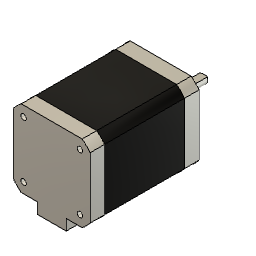
Planetary Gear Module v11 (Autodesk Fusion 360 archive; units mm, degrees)
design "Nema 17 Stepper Motor 60mm"
Autodesk Fusion 360 part; units mm, degrees
sketch "Sketch1" plane through (0, 0, 0) normal (0, 0, 1) x (1, 0, 0)
  line L0 (-15.5, 15.5) -> (15.5, 15.5) construction
  line L1 (15.5, 15.5) -> (15.5, -15.5) construction
  line L2 (15.5, -15.5) -> (-15.5, -15.5) construction
  line L3 (-15.5, -15.5) -> (-15.5, 15.5) construction
  line L4 (15.5, 15.5) -> (-15.5, -15.5) construction
  line L5 (-21.15, 21.15) -> (21.15, 21.15)
  line L6 (21.15, 21.15) -> (21.15, -21.15)
  line L7 (21.15, -21.15) -> (-21.15, -21.15)
  line L8 (-21.15, -21.15) -> (-21.15, 21.15)
  line L9 (-21.15, 21.15) -> (21.15, -21.15) construction
  arc A0 (-21.15, -16.7833) -> (-16.7833, -21.15) centre (0, 0) ccw
  arc A1 (16.7833, -21.15) -> (21.15, -16.7833) centre (0, 0) ccw
  arc A2 (21.15, 16.7833) -> (16.7833, 21.15) centre (0, 0) ccw
  arc A3 (-16.7833, 21.15) -> (-21.15, 16.7833) centre (0, 0) ccw
  circle A4 centre (0, 0) radius 11
  circle A5 centre (0, 0) radius 2.5
  line L10 (-2, 1.5) -> (2, 1.5)
  circle A6 centre (-15.5, 15.5) radius 1.5
  circle A7 centre (-15.5, -15.5) radius 1.5
  circle A8 centre (15.5, -15.5) radius 1.5
  circle A9 centre (15.5, 15.5) radius 1.5
  circle A10 centre (0, 0) radius 5
  line L11 (0, -2.5) -> (0, 1.5) construction
  line L12 (8, -21.15) -> (8, -27.15)
  line L13 (8, -27.15) -> (-8, -27.15)
  line L14 (-8, -27.15) -> (-8, -21.15)
  line L15 (0, 0) -> (0, -21.15) construction
  point P0 (0, -2.5)
  dimension "d37" = 60
  dimension "d39" = -52
  dimension "d40" = 0
  constraint horizontal L0
  constraint vertical L1
  constraint horizontal L2
  constraint vertical L3
  constraint equal L0 L3
  constraint midpoint A0.centre L4
  constraint coincident A0.centre A1.centre
  constraint horizontal L5
  constraint vertical L6
  constraint horizontal L7
  constraint vertical L8
  constraint coincident L4 L7.end
  constraint coincident L4 L5.end
  constraint coincident L8 A3.end
  constraint coincident L8 A0.start
  constraint coincident L7 A0.end
  constraint concentric A0 A1
  constraint coincident L7 A1.start
  constraint coincident L6 A1.end
  constraint coincident L6 A2.start
  constraint coincident L5 A3.start
  constraint concentric A2 A3
  constraint coincident L5 A2.end
  constraint equal A2 A3
  constraint equal A1 A3
  constraint equal A0 A3
  constraint concentric A2 A4
  constraint coincident A5 L10.start
  constraint coincident A5 L10.end
  constraint horizontal L10
  constraint coincident A5 P0
  constraint coincident L0.start L3.end
  constraint concentric A0 A10
  constraint midpoint A0.centre L9
  constraint coincident P0 L11.start
  constraint midpoint L10 L11.end
  constraint vertical L11
  constraint symmetric L12.end L13.end L15
  constraint perpendicular L12 L13
  constraint midpoint L7 L15.end
  constraint coincident L7 L14.end
  constraint perpendicular L7 L14
  constraint coincident L7 L12.start
  measures "d1" distance of L0.start L0.end
  measures "d3" distance of A0.centre L0.end
  measures "d7" distance of L5.start L5.end
  measures "d16" diameter of A0
  measures "d17" diameter of A4
  measures "d18" diameter of A5
  measures "d19" distance of L10 P0
  measures "d20" diameter of A6
  measures "d23" diameter of A10
  measures "d70" distance of L12.end L13.end
  measures "d230" distance of L12.start L12.end
ref_plane "WorkPlane1" through (0, 0, -12) normal (0, 0, 1) x (1, 0, 0)
extrude "Extrude6" add sketch "Sketch1" along normal blind 60 and the other way blind -52 contours L5 L6 L7 L8 A0 A1 A2 A3 | L7 L12 L13 L14 | A4 | A5 L10 | A5 L10 | A10 makes body 1
extrude "Extrude5" add sketch "Sketch1" along normal blind 52 and the other way blind -8 separate body contours L5 L6 L7 L8 A0 A1 A2 A3 | A4 | A5 L10 | A5 L10 | A6 | A7 | A8 | A9 | A10 makes body 2
extrude "Extrude1" add sketch "Sketch1" along normal blind 8 separate body contours L5 L6 L7 L8 A0 A1 A2 A3 | A4 | A5 L10 | A5 L10 | A10 makes body 3
extrude "Extrude2" add sketch "Sketch1" against normal blind 2 contours A4 bodies 3
extrude "Extrude1'" add sketch "Sketch1" against normal blind 27 separate body contours A5 L10 picked at (-0.6617, 0.293) makes body 4 in component "27mm Shaft"
extrude "Extrude2'" add sketch "Sketch1" against normal blind 12 contours A5 L10 picked at (0.0594, 2.0106) bodies 4 in component "27mm Shaft"
chamfer "Chamfer1" distance 0.5 angle 45 1 edges at (0, -2.5, -27) on bodies 4 in component "27mm Shaft"
extrude "Extrude1''" add sketch "Sketch1" against normal blind 24 separate body contours A5 L10 picked at (-0.6617, 0.293) makes body 5 in component "24mm Shaft"
extrude "Extrude2''" add sketch "Sketch1" against normal blind 9 contours A5 L10 picked at (0.0594, 2.0106) bodies 5 in component "24mm Shaft"
chamfer "Chamfer1'" distance 0.5 angle 45 1 edges at (0, -2.5, -24) on bodies 5 in component "24mm Shaft"
component "27mm Shaft" placed x (1, 0, 0) y (0, 1, 0) z (0, 0, 1) at (0, 0, 0)
component "24mm Shaft" placed x (1, 0, 0) y (0, 1, 0) z (0, 0, 1) at (0, 0, 0)
equation "d22 = 360.0 °"
equation "d36 = 0.0 °"
equation "d40 = 0.0 °"
equation "d347 = 15 mm - 27 mm"
equation "d352 = 15 mm - 24 mm"
equation "d31 = -27 mm + 15 mm"
equation "d67 = ( -( 15 - 7 ) / 2 ) * 1 mm"
equation "d75 = 140 mm"
equation "d112 = d75 + 12 mm"
equation "d126 = 7 mm - 84.00 mm"

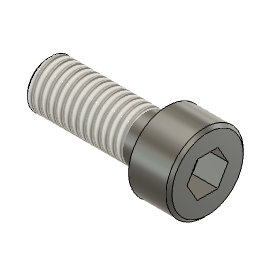
design "M8 x 20mm Cap Screw"
Autodesk Fusion 360 part; units mm, degrees
cylinder "CylinderPrimitive1" add diameter 13 height 6.8 placed x (0, 0, -1) y (0, 1, 0) z (1, 0, 0) at (0, 0, 0)
sketch "Sketch2" plane through (6.8, 0, 0) normal (1, 0, 0) x (0, 0, -1)
  circle A0 centre (0, 0) radius 6.5
  line L0 (1.7321, -3) -> (3.4641, 0)
  line L1 (3.4641, 0) -> (1.7321, 3)
  line L2 (1.7321, 3) -> (-1.7321, 3)
  line L3 (-1.7321, 3) -> (-3.4641, 0)
  line L4 (-3.4641, 0) -> (-1.7321, -3)
  line L5 (-1.7321, -3) -> (1.7321, -3)
  dimension "d3" = 6
  constraint coincident A0.centre origin
  constraint horizontal L5
  measures "d3" distance of L2 L5
extrude "Extrude1" cut sketch "Sketch2" against normal blind 4.3 contours L0 L1 L2 L3 L4 L5
chamfer "Chamfer1" distance 0.5 angle 45 1 edges at (6.8, -2.3505, 6.0601)
cylinder "CylinderPrimitive2" add diameter 8 height 20 placed x (0, 0, 1) y (0, 1, 0) z (-1, 0, 0) at (0, 0, 0)
chamfer "Chamfer2" distance 0.5 angle 45 1 edges at (-20, -1.4465, -3.7293)
thread "Thread1" "ISO Metric profile 8.0 M8x1.25 6g" major diameter 7.866 minor diameter 6.4455 pitch 1.25 angle 60 resizes the face on face at (-13, -0.3983, 3.9801) from (-3.5, 0, 0) to (-19.5, 0, 0)
